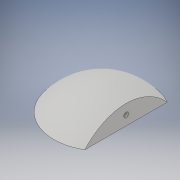
# Autodesk Inventor part: camera side
Saved by Autodesk Inventor 2017 (Build 210142000, 142)
## iProperties
Created: 2020-02-20
Part Number: camera side
Material: Generic
Document SubType Name: Modeling
Designer: S346852600
Density: 1 g/cm^3
Appearance: Default
Author: S346852600
Autodesk Inventor part; units mm, degrees
ref_plane "YZ Plane" through (0, 0, 0) normal (1, 0, 0) x (0, 1, 0)
ref_plane "XZ Plane" through (0, 0, 0) normal (0, 1, 0) x (-1, 0, 0)
ref_plane "XY Plane" through (0, 0, 0) normal (0, 0, 1) x (1, 0, 0)
sketch "Sketch1" plane through (0, 0, 0) normal (1, 0, 0) x (0, 1, 0)
  line L0 (0, 0) -> (0, 25.4)
  line L1 (0, 0) -> (13.97, 0)
  arc A0 (13.97, 0) -> (0, 25.4) centre (-21.4675, -2.9489) ccw
  line L2 (0, 0) -> (0, 15.748)
  line L3 (0, 15.748) -> (8.7805, 15.748)
  dimension "d0" = 25.4
  dimension "d1" = 13.97
  dimension "d2" = 35.56
  dimension "d3" = 15.748
  constraints: 8 end point, 3 point on circle, 1 centre point, 1 horizontal, 1 perpendicular, 1 point on line, 1 vertical
  measures "d0" distance of L0.start L0.end
  measures "d1" distance of L0.start L1.end
  measures "d2" radius of A0
  measures "d3" distance of L0.start L2.end
revolve "Revolution1" add sketch "Sketch1" angle 360 about axis through (0, 0, 0) along (0, 1, 0)
sketch "Sketch4" plane through (0, 0, 0) normal (0, -1, 0) x (1, 0, 0)
  line L0 (0, 0) -> (12.897, 0)
  line L1 (12.897, 0) -> (12.897, 21.8821)
  circle A0 centre (0, 0) radius 25.4 projected
  line L2 (12.897, 21.8821) -> (38.6124, 21.8821)
  line L3 (38.6124, 21.8821) -> (38.6124, -32.9808)
  line L4 (38.6124, -32.9808) -> (12.897, -32.9808)
  line L5 (12.897, -32.9808) -> (12.897, 21.8821)
  dimension "d12" = 21.8821
  constraints: 12 end point, 2 horizontal, 2 parallel, 1 perpendicular, 1 vertical, 2 other
  measures "d12" distance of L0.end L1.end
extrude "Extrusion3" cut sketch "Sketch4" against normal through all contours L1 A0 L5 | L2 L3 L4 L5 A0 picked at (14.3084, 13.5451)
sketch "Sketch5" plane through (12.897, 0, 21.8821) normal (1, 0, 0) x (0, 0, -1)
  line L0 (21.8821, 0) -> (21.8821, 5.08)
  circle A0 centre (21.8821, 5.08) radius 1.27
  dimension "d15" = 5.08
  dimension "d16" = 2.54
  constraints: 2 end point, 1 centre point, 1 coincident, 1 vertical
  measures "d15" distance of L0.start L0.end
  measures "d16" diameter of A0
extrude "Extrusion4" cut sketch "Sketch5" against normal blind 2.54
sketch "Sketch6" plane through (0, 0, 0) normal (0, -1, 0) x (1, 0, 0)
  circle A0 centre (0, 0) radius 1.27
  dimension "d19" = 2.54
  constraints: 1 centre point, 1 coincident
  measures "d19" diameter of A0
extrude "Extrusion5" cut sketch "Sketch6" against normal blind 2.54
body "Solid1"
